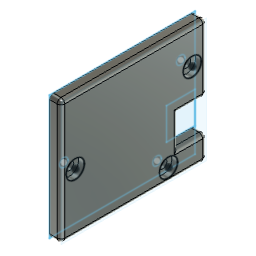
Cover_v1 v2 (Autodesk Fusion 360 design; units mm, degrees)
Autodesk Fusion 360 part; units mm, degrees
sketch "Sketch1" plane through (0, 0, 0) normal (1, 0, 0) x (0, 1, 0)
  line L0 (-19.1488, 16.2315) -> (19.1512, 16.2315)
  line L1 (19.1512, 16.2315) -> (19.1512, -16.3685)
  line L2 (19.1512, -16.3685) -> (-19.1488, -16.3685)
  line L3 (-19.1488, -16.3685) -> (-19.1488, 16.2315)
  circle A0 centre (-15.3988, -0.9685) radius 1.1
  circle A1 centre (15.4012, 6.9815) radius 1.1
  circle A2 centre (9.1512, -12.8825) radius 1.1
  line L4 (19.1512, -9.8685) -> (11.6512, -9.8685)
  line L5 (11.6512, -9.8685) -> (11.6512, -1.5685)
  line L6 (11.6512, -1.5685) -> (19.1512, -1.5685)
  line L7 (19.1512, -1.5685) -> (19.1512, -9.8685)
  dimension "d1" = 38.3
  dimension "d2" = 32.6
  dimension "d3" = 2.2
  dimension "d4" = 15.4
  dimension "d5" = 3.75
  dimension "d6" = 2.2
  dimension "d7" = 9.25
  dimension "d8" = 3.75
  dimension "d9" = 2.2
  dimension "d10" = 10
  dimension "d11" = 3.486
  dimension "d23" = 7.5
  dimension "d24" = 8.3
  dimension "d25" = 6.5
  constraint horizontal L0
  constraint vertical L1
  constraint horizontal L2
  constraint vertical L3
  constraint horizontal L4
  constraint vertical L5
  constraint horizontal L6
  constraint vertical L7
  constraint coincident L1 L4.start
  measures "d1" distance of L0.start L0.end
  measures "d2" distance of L0.start L2.end
  measures "d3" diameter of A0
  measures "d4" distance of L2 A0.centre
  measures "d5" distance of L3 A0.centre
  measures "d6" diameter of A1
  measures "d7" distance of L0 A1.centre
  measures "d8" distance of L1 A1.centre
  measures "d9" diameter of A2
  measures "d10" distance of L1 A2.centre
  measures "d11" distance of L2 A2.centre
  measures "d23" distance of L4.start L4.end
  measures "d24" distance of L4.start L6.end
  measures "d25" distance of L2 L4
extrude "Extrude1" add sketch "Sketch1" along normal blind 3
sketch "Sketch2" plane through (3, 0, 0) normal (1, 0, 0) x (0, 1, 0)
  circle A0 centre (9.1512, -12.8825) radius 1.1
  circle A1 centre (15.4012, 6.9815) radius 1.1
  circle A2 centre (-15.3988, -0.9685) radius 1.1
  line L0 (-19.1488, -16.3685) -> (19.1512, -16.3685)
  line L1 (19.1512, -16.3685) -> (19.1512, 16.2315)
  line L2 (19.1512, 16.2315) -> (-19.1488, 16.2315)
  line L3 (-19.1488, 16.2315) -> (-19.1488, -16.3685)
  circle A3 centre (-15.3988, -0.9685) radius 2.4
  circle A4 centre (9.1512, -12.8825) radius 2.4
  circle A5 centre (15.4012, 6.9815) radius 2.4
  dimension "d14" = 4.8
  dimension "d15" = 4.8
  dimension "d16" = 4.8
  constraint concentric A2 A3
  constraint concentric A0 A4
  constraint concentric A1 A5
  measures "d14" diameter of A3
  measures "d15" diameter of A4
  measures "d16" diameter of A5
extrude "Extrude2" cut sketch "Sketch2" against normal blind 1.5 contours A3
extrude "Extrude3" cut sketch "Sketch2" against normal blind 1.5 contours A4
extrude "Extrude4" cut sketch "Sketch2" against normal blind 1.5 contours A5
extrude "Extrude5" cut sketch "Sketch1" along normal blind 3 contours L1 L4 L5 L6 L7
fillet "Fillet1" radius 1 1 edges at (3, 0.0012, 16.2315)
fillet "Fillet2" radius 1 3 edges at (1, -19.1488, 16.2315) (2.7071, -19.1488, 15.9387) (3, -19.1488, -0.5685)
fillet "Fillet3" radius 1 3 edges at (1, -19.1488, -16.3685) (2.7071, -18.856, -16.3685) (3, 0.5012, -16.3685)
fillet "Fillet4" radius 1 3 edges at (1, 19.1512, -16.3685) (2.7071, 19.1512, -16.0756) (3, 19.1512, -12.6185)
fillet "Fillet5" radius 1 3 edges at (1, 19.1512, -9.8685) (2.7071, 18.8583, -9.8685) (3, 14.9012, -9.8685)
fillet "Fillet6" radius 1 1 edges at (3, 11.6512, -6.2185)
fillet "Fillet7" radius 1 1 edges at (3, 14.9012, -1.5685)
fillet "Fillet8" radius 1 5 edges at (1, 19.1512, -1.5685) (2.7071, 19.1512, -1.2756) (3, 19.1512, 7.3315) (2.7071, 19.1512, 15.9387) (1, 19.1512, 16.2315)
